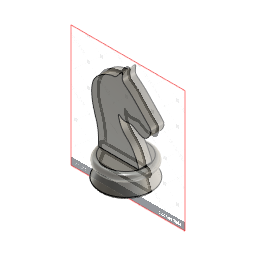
chess v2 (Autodesk Fusion 360 design; units mm, degrees)
Autodesk Fusion 360 part; units mm, degrees
sketch "Sketch9" plane through (0, 0, 0) normal (0, 1, 0) x (1, 0, 0)
  spline S0 degree 5 poles (-3.0245, -3.5245) (-3.0369, -3.5369) (-3.0513, -3.5718) (-3.0497, -3.6631) (-3.035, -3.8911) (-3.0329, -4.3447) (-3.0679, -4.9265) (-3.1413, -5.5713) (-3.2456, -6.213) (-3.3699, -6.8028) (-3.5055, -7.3236) (-3.6444, -7.7794) (-3.7792, -8.1891) (-3.9021, -8.5798) (-4.0047, -8.979) (-4.0773, -9.4083) (-4.1086, -9.8755) (-4.0867, -10.3777) (-4.0011, -10.9033) (-3.8445, -11.435) (-3.6137, -11.9521) (-3.3119, -12.4331) (-2.9502, -12.8587) (-2.547, -13.2134) (-2.1252, -13.4873) (-1.7088, -13.6778) (-1.3205, -13.7915) (-0.9787, -13.845) (-0.6946, -13.8683) (-0.4701, -13.9009) (-0.2975, -13.979) (-0.1588, -14.125) (-0.0244, -14.3356) (0.1315, -14.5849) (0.319, -14.8285) (0.5116, -15.0036) (0.6531, -15.0441) (0.6996, -14.9107) (0.6642, -14.6278) (0.6079, -14.2699) (0.6015, -13.9222) (0.7, -13.6525) (0.9049, -13.4714) (1.179, -13.346) (1.4723, -13.2254) (1.7439, -13.0614) (1.9874, -12.8335) (2.2202, -12.5417) (2.4711, -12.1996) (2.7683, -11.8263) (3.1279, -11.4395) (3.5399, -11.0469) (3.9732, -10.6482) (4.3844, -10.2399) (4.7261, -9.8191) (4.955, -9.3876) (5.0397, -8.9558) (4.97, -8.5475) (4.7633, -8.2023) (4.454, -7.9627) (4.0845, -7.8608) (3.6954, -7.9076) (3.3146, -8.0762) (2.9546, -8.3062) (2.6177, -8.5273) (2.299, -8.6783) (1.9902, -8.7248) (1.6831, -8.6849) (1.373, -8.6246) (1.0603, -8.6171) (0.7526, -8.7144) (0.4676, -8.9081) (0.233, -9.1152) (0.0762, -9.2319) (0.0184, -9.17) (0.0639, -8.9101) (0.202, -8.4935) (0.413, -7.9931) (0.6723, -7.4907) (0.9555, -7.0534) (1.2433, -6.7048) (1.5238, -6.4244) (1.7901, -6.1693) (2.0404, -5.8905) (2.2766, -5.5495) (2.5037, -5.1375) (2.728, -4.6887) (2.9495, -4.2582) (3.1514, -3.9032) (3.2976, -3.6647) (3.3111, -3.5427) (3.099, -3.4909) (2.6647, -3.4816) (2.048, -3.4895) (1.3203, -3.4988) (0.5515, -3.5018) (-0.1979, -3.4981) (-0.9276, -3.5031) (-1.6138, -3.5148) (-2.2077, -3.5212) (-2.6607, -3.5121) (-2.8862, -3.499) (-2.9772, -3.4977) (-3.0121, -3.5121) (-3.0245, -3.5245) knots 0 0 0 0 0 0 0.01 0.02 0.03 0.04 0.05 0.06 0.07 0.08 0.09 0.1 0.11 0.12 0.13 0.14 0.15 0.16 0.17 0.18 0.19 0.2 0.21 0.22 0.23 0.24 0.25 0.26 0.27 0.28 0.29 0.3 0.31 0.32 0.33 0.34 0.35 0.36 0.37 0.38 0.39 0.4 0.41 0.42 0.43 0.44 0.45 0.46 0.47 0.48 0.49 0.5 0.51 0.52 0.53 0.54 0.55 0.56 0.57 0.58 0.59 0.6 0.61 0.62 0.63 0.64 0.65 0.66 0.67 0.68 0.69 0.7 0.71 0.72 0.73 0.74 0.75 0.76 0.77 0.78 0.79 0.8 0.81 0.82 0.83 0.84 0.85 0.86 0.87 0.88 0.89 0.9 0.91 0.92 0.93 0.94 0.95 0.96 0.97 0.98 0.99 1 1 1 1 1 1
  line L0 (3.1772, -4.0545) -> (3.3772, -3.2545)
  line L1 (2.4, -3.5) -> (-2.4, -3.5)
  line L2 (-2.8245, -3.3245) -> (-3.2245, -3.7245)
  point P0 (-3.2208, -6.0333)
  point P1 (-4, -9)
  point P2 (-3.4561, -12.1845)
  point P3 (-1.1337, -13.8164)
  point P4 (-0.3, -14)
  point P5 (0.2471, -14.7266)
  point P6 (0.6551, -14.9776)
  point P7 (0.6394, -13.8792)
  point P8 (1.4868, -13.2045)
  point P9 (2.852, -11.7451)
  point P10 (5, -9)
  point P11 (3.9, -7.9)
  point P12 (2.138, -8.6908)
  point P13 (0.8434, -8.7009)
  point P14 (0.0745, -9.1874)
  point P15 (0.7976, -7.3098)
  point P16 (2.2451, -5.5787)
  point P17 (3.2772, -3.6545)
  point P18 (0, -3.5)
  constraint midpoint P17 L0
  constraint midpoint P18 L1
  constraint midpoint S0.start L2
sketch "Sketch10" plane through (0, 0, 0) normal (0, 1, 0) x (1, 0, 0)
  line L0 (-3, -3.5) -> (0, -3.5)
  line L1 (0, -3.5) -> (0, -1.9)
  line L2 (0, -1.9) -> (-3, -1.9)
  arc A0 (-3, -1.9) -> (-3, -3.5) centre (-3, -2.7) ccw
  constraint horizontal L0
  constraint vertical L1
  constraint horizontal L2
  constraint tangent L2 A0
sketch "Sketch11" plane through (0, 0, 0) normal (0, 1, 0) x (1, 0, 0)
  line L0 (-3, -2) -> (0.001, -2)
  line L1 (0.001, 0) -> (-3, 0)
  line L2 (-3, -2) -> (-3.8191, -0.3618)
  line L3 (-3.5955, 0) -> (-3, 0)
  arc A0 (-3.5955, 0) -> (-3.8191, -0.3618) centre (-3.5955, -0.25) ccw
  line L4 (0.001, -2) -> (0.001, 0)
  dimension "d11" = 0.25
  constraint horizontal L0
  constraint horizontal L1
  constraint tangent L2 A0
  constraint tangent L3 A0
  constraint perpendicular L1 L4
  measures "d11" radius of A0
sketch "Sketch12" plane through (0, 0, 0) normal (1, 0, 0) x (0, 1, 0)
sketch "Sketch15" plane through (0, 0, 0) normal (0, 1, 0) x (1, 0, 0)
  line L0 (-3, -3.5) -> (0, -3.5)
  line L1 (0, -3.5) -> (0, -2)
  line L2 (0, -2) -> (-3, -2)
  arc A0 (-3, -2) -> (-3, -3.5) centre (-3, -2.75) ccw
  line L3 (-3, -2) -> (0, -2)
  line L4 (0, -2) -> (0, 0)
  line L5 (0, 0) -> (-3, 0)
  line L6 (-3, -2) -> (-3.6534, -0.2535)
  line L7 (-3.4742, 0.003) -> (-3, 0)
  arc A1 (-3.4742, 0.003) -> (-3.6534, -0.2535) centre (-3.4754, -0.187) ccw
  dimension "d17" = 0.19
  constraint horizontal L0
  constraint vertical L1
  constraint horizontal L2
  constraint horizontal L3
  constraint vertical L4
  constraint horizontal L5
  constraint coincident L4.end L5.start
  constraint tangent L6 A1
  constraint tangent L7 A1
  measures "d17" radius of A1
sketch "Sketch16" plane through (0, 0, 0) normal (0, 1, 0) x (1, 0, 0)
  line L0 (30.01, -50.1207) -> (0.01, -50.1207)
  line L1 (0.01, -50.1207) -> (0.01, -0.1207)
  line L2 (0.01, -0.1207) -> (30.01, -0.1207)
  line L3 (30.01, -0.1207) -> (30.01, -50.1207)
  dimension "d21" = 30
  dimension "d22" = 50
  constraint horizontal L0
  constraint vertical L1
  constraint horizontal L2
  constraint vertical L3
  measures "d21" distance of L0.start L0.end
  measures "d22" distance of L0.start L2.end
sketch "Sketch17" plane through (0, 0, 0) normal (0, 1, 0) x (1, 0, 0)
  spline S0 degree 5 poles (-9.5358, -11.0085) (-9.5628, -11.0594) (-9.5847, -11.198) (-9.5475, -11.5409) (-9.469, -12.3478) (-9.4298, -13.8318) (-9.4992, -15.5839) (-9.6659, -17.3451) (-9.9049, -18.9258) (-10.1984, -20.2786) (-10.5338, -21.4513) (-10.8996, -22.5487) (-11.2833, -23.6915) (-11.6683, -24.9769) (-12.0307, -26.437) (-12.3408, -28.0528) (-12.5648, -29.7712) (-12.6658, -31.5207) (-12.6057, -33.2276) (-12.3468, -34.8311) (-11.8523, -36.3023) (-11.0947, -37.6368) (-10.0663, -38.8414) (-8.789, -39.9214) (-7.3236, -40.8701) (-5.7812, -41.6529) (-4.3315, -42.202) (-3.1571, -42.4486) (-2.3026, -42.5066) (-1.7248, -42.5469) (-0.8744, -43.4013) (0.277, -44.9112) (1.2765, -46.1298) (1.6705, -46.1484) (1.5453, -45.146) (1.4174, -44.1003) (1.4238, -43.1917) (1.6674, -42.4981) (2.1668, -41.9002) (2.9422, -41.2749) (3.9839, -40.477) (5.2646, -39.4024) (6.7324, -38.0145) (8.3121, -36.3915) (9.9105, -34.686) (11.4252, -33.0704) (12.7521, -31.6953) (13.7924, -30.6244) (14.4626, -29.8224) (14.6957, -29.0188) (14.4667, -27.867) (13.8316, -26.5516) (12.8835, -25.3881) (11.7342, -24.737) (10.4832, -24.7644) (9.1996, -25.3407) (7.9296, -26.1807) (6.7004, -26.9513) (5.5254, -27.3867) (4.4084, -27.4124) (3.3496, -27.2293) (2.3533, -27.1309) (1.437, -27.3584) (0.64, -27.9259) (0.029, -28.5002) (-0.3294, -28.6572) (-0.3972, -28.1339) (-0.1846, -27.0108) (0.2694, -25.5456) (0.9101, -24.0557) (1.6826, -22.7865) (2.5477, -21.7741) (3.4772, -20.9069) (4.4478, -20.0022) (5.4354, -18.8817) (6.4096, -17.4376) (7.3271, -15.726) (8.1291, -13.9692) (8.7466, -12.446) (9.1011, -11.3844) (9.1127, -10.9073) (8.6915, -10.8302) (7.7745, -10.8617) (6.3602, -10.9058) (4.4926, -10.9145) (2.2636, -10.9045) (-0.1926, -10.9049) (-2.7012, -10.9348) (-5.0505, -10.9676) (-7.0352, -10.9699) (-8.4892, -10.9221) (-9.1704, -10.8812) (-9.4225, -10.8926) (-9.5087, -10.9576) (-9.5358, -11.0085) knots 0 0 0 0 0 0 0.01111111 0.02222222 0.03333333 0.04444444 0.05555556 0.06666667 0.07777778 0.08888889 0.1 0.11111111 0.12222222 0.13333333 0.14444444 0.15555556 0.16666667 0.17777778 0.18888889 0.2 0.21111111 0.22222222 0.23333333 0.24444444 0.25555556 0.26666667 0.27777778 0.28888889 0.3 0.31111111 0.32222222 0.33333333 0.34444444 0.35555556 0.36666667 0.37777778 0.38888889 0.4 0.41111111 0.42222222 0.43333333 0.44444444 0.45555556 0.46666667 0.47777778 0.48888889 0.5 0.51111111 0.52222222 0.53333333 0.54444444 0.55555556 0.56666667 0.57777778 0.58888889 0.6 0.61111111 0.62222222 0.63333333 0.64444444 0.65555556 0.66666667 0.67777778 0.68888889 0.7 0.71111111 0.72222222 0.73333333 0.74444444 0.75555556 0.76666667 0.77777778 0.78888889 0.8 0.81111111 0.82222222 0.83333333 0.84444444 0.85555556 0.86666667 0.87777778 0.88888889 0.9 0.91111111 0.92222222 0.93333333 0.94444444 0.95555556 0.96666667 0.97777778 0.98888889 1 1 1 1 1 1
  line L0 (9.6399, -11.8377) -> (8.3601, -10.1623)
  line L1 (-9, -10) -> (-10.0715, -12.017)
  line L2 (13.373, -32.2135) -> (15.5162, -27.049)
  line L3 (1.1123, -47.7191) -> (2, -44)
  line L4 (-5, -41) -> (1.4282, -44.3389)
  point P0 (-9.6564, -17.065)
  point P1 (-11.2997, -23.7782)
  point P2 (-12.5165, -33.5542)
  point P3 (-7, -41)
  point P4 (-1.7859, -42.6695)
  point P5 (1.5561, -45.8596)
  point P6 (1.591, -42.8233)
  point P7 (5.4832, -39.1695)
  point P8 (14.4446, -29.6312)
  point P9 (12, -25)
  point P10 (5.714, -27.2467)
  point P11 (1.5602, -27.4005)
  point P12 (-0.209, -28.5159)
  point P13 (1, -24)
  point P14 (6, -18)
  point P15 (9, -11)
  point P16 (-0.1013, -10.9113)
  constraint midpoint P15 L0
  constraint midpoint S0.start L1
  constraint midpoint P8 L2
  constraint midpoint P5 L3
  constraint midpoint P4 L4
extrude "Extrude3" add sketch "Sketch17" along normal blind 6
move_body "Move4" bodies 1 to x (1, 0, 0) y (0, 1, 0) z (0, 0, 1) at (-0.0221, -2.6468, -0.0665)
sketch "Sketch18" plane through (0, 0, 0) normal (0, 1, 0) x (1, 0, 0)
  line L0 (-9.5771, -11) -> (0, -11)
  line L1 (0, -11) -> (0, -7)
  line L2 (0, -7) -> (-9.5771, -7)
  arc A0 (-9.5771, -7) -> (-9.5771, -11) centre (-9.5771, -9) ccw
  line L3 (-9.5771, -7) -> (0, -7)
  line L4 (0, -7) -> (0, -1.5)
  line L5 (0, -1.5) -> (-9.5771, -1.5)
  line L6 (-9.5771, -7) -> (-11.6909, -2.2016)
  line L7 (-11.2334, -1.5) -> (-9.5771, -1.5)
  arc A1 (-11.2334, -1.5) -> (-11.6909, -2.2016) centre (-11.2334, -2) ccw
  dimension "d25" = 0.5
  constraint horizontal L0
  constraint vertical L1
  constraint horizontal L2
  constraint tangent L2 A0
  constraint horizontal L3
  constraint vertical L4
  constraint horizontal L5
  constraint tangent L6 A1
  constraint tangent L7 A1
  measures "d25" radius of A1
move_body "Move5" bodies 1 to x (1, 0, 0) y (0, 1, 0) z (0, 0, 1) at (0, -0.4145, 0)
revolve "Revolve4" add sketch "Sketch18" angle 360 about axis through (0, 0, 7) along (0, 0, -1)
